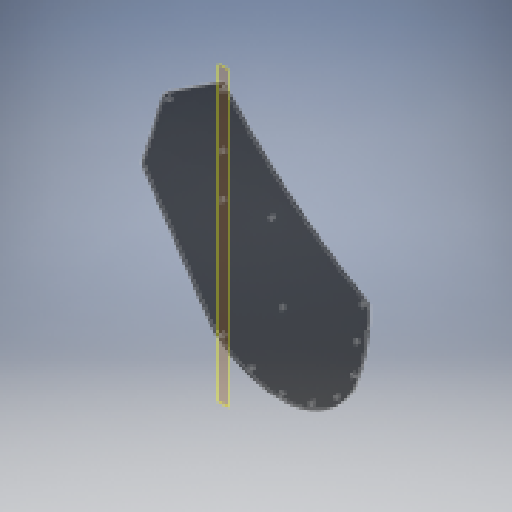
# Autodesk Inventor part: PolyIntakeSides
Saved by Autodesk Inventor 2026.1 (Build 301233000, 233)
## iProperties
Created: 2025-09-20
Part Number: PolyIntakeSides
Material: Polycarbonate, Smoke
Document SubType Name: Modeling
Designer: Teddy
Density: 1.2 g/cm^3
Appearance: Polycarbonate - Smoked
Author: Teddy
Autodesk Inventor part; units mm, degrees
ref_plane "YZ Plane" through (0, 0, 0) normal (1, 0, 0) x (0, 1, 0)
ref_plane "XZ Plane" through (0, 0, 0) normal (0, 1, 0) x (-1, 0, 0)
ref_plane "XY Plane" through (0, 0, 0) normal (0, 0, 1) x (1, 0, 0)
ref_plane "Work Plane1" through (0, 0, 0) normal (0, 0, 1) x (1, 0, 0)
sketch "Sketch1" plane through (0, 0, 0) normal (0, 0, 1) x (1, 0, 0)
  circle A0 centre (1.1684, 152.4) radius 2.0828 projected
  circle A1 centre (1.1684, 88.9) radius 2.1844 projected
  circle A2 centre (1.1684, 38.1) radius 2.1844 projected
  circle A3 centre (61.0614, 49.4192) radius 2.1844 projected
  circle A4 centre (1.1684, -101.6) radius 2.1844 projected
  circle A5 centre (169.7176, 13.9463) radius 2.1844 projected
  circle A6 centre (-62.568, 110.6374) radius 2.1844 projected
  arc A7 (-66.0482, 115.9488) -> (-68.6382, 112.5014) centre (-62.568, 110.6374) ccw
  arc A8 (5.9747, 156.5499) -> (-2.3118, 157.7114) centre (1.1684, 152.4) ccw
  arc A9 (171.6835, 7.9082) -> (176.0627, 14.1942) centre (169.7176, 13.9463) ccw construction
  circle A10 centre (61.0614, 49.4192) radius 6.35 construction
  circle A11 centre (1.1684, 88.9) radius 6.35 construction
  circle A12 centre (1.1684, 38.1) radius 6.35 construction
  arc A13 (-3.0452, -106.3506) -> (-2.7826, -106.5711) centre (1.1684, -101.6) ccw
  line L0 (-66.0482, 115.9488) -> (-2.3118, 157.7114)
  arc A14 (5.9747, 156.5499) -> (172.8551, 19.467) centre (486.6085, 571.5392) ccw
  circle A15 centre (72.9495, -37.5108) radius 2.286
  line L1 (-82.8745, 72.8532) -> (22.0714, -87.311) construction
  line L2 (-72.2491, -17.1807) -> (-105.9376, 34.2333) construction
  arc A16 (171.6835, 7.9082) -> (153.2328, 1.3335) centre (281.7757, -330.2205) ccw construction
  arc A17 (10.0948, -100.7846) -> (6.0913, -105.6109) centre (281.7757, -330.2205) ccw construction
  arc A18 (19.0893, -100.0694) -> (10.0948, -100.7846) centre (14.9463, -104.8817) ccw construction
  arc A19 (153.2328, 1.3335) -> (149.6297, -6.9388) centre (155.5282, -4.5871) ccw construction
  line L3 (12.9609, -192.1214) -> (40.8456, -173.8503) construction
  arc A20 (19.0893, -100.0694) -> (38.9783, -112.7468) centre (72.9495, -37.5108) ccw construction
  line L4 (281.7757, -330.2205) -> (72.9495, -37.5108) construction
  line L5 (40.8456, -173.8503) -> (129.0057, -116.0843) construction
  arc A21 (36.3651, -118.5342) -> (161.4679, -29.2829) centre (72.9495, -37.5108) ccw construction
  arc A22 (33.752, -124.3216) -> (75.4374, -132.7283) centre (72.9495, -37.5108) ccw construction
  arc A23 (39.5647, -113.0492) -> (33.752, -124.3216) centre (36.3651, -118.5342) ccw construction
  arc A24 (167.7906, -28.6951) -> (155.4015, -31.1592) centre (161.4679, -29.2829) ccw construction
  arc A25 (38.9783, -112.7468) -> (155.1451, -29.8706) centre (72.9495, -37.5108) ccw construction
  arc A26 (155.1451, -29.8706) -> (149.6297, -6.9388) centre (72.9495, -37.5108) ccw construction
  arc A27 (161.8616, -71.6749) -> (176.0627, 14.1942) centre (-39.6726, 5.7638) ccw
  arc A28 (161.8616, -71.6749) -> (167.7906, -28.6951) centre (72.9495, -37.5108) ccw construction
  arc A29 (176.0627, 14.1942) -> (172.8551, 19.467) centre (169.7176, 13.9463) ccw
  arc A30 (-2.7826, -106.5711) -> (75.4374, -132.7283) centre (72.286, -12.1194) ccw
  arc A31 (75.4374, -132.7283) -> (161.8616, -71.6749) centre (72.9495, -37.5108) ccw
  arc A32 (-2.7826, -106.5711) -> (6.0913, -105.6109) centre (1.1684, -101.6) ccw construction
  circle A33 centre (36.3651, -118.5342) radius 2.286
  circle A34 centre (72.4832, -126.4095) radius 2.286
  circle A35 centre (108.6819, -118.9135) radius 2.286
  circle A36 centre (138.7021, -97.3421) radius 2.286
  circle A37 centre (157.3531, -65.4254) radius 2.286
  circle A38 centre (161.41, -28.682) radius 2.286
  line L6 (-68.6382, 112.5014) -> (-92.7323, 34.0383)
  line L7 (-91.2146, 23.3498) -> (-16.2187, -91.1058)
  arc A39 (-16.2187, -91.1058) -> (-3.0452, -106.3506) centre (47.5176, -49.3432) ccw
  line L8 (-82.8745, 72.8532) -> (-83.8065, 69.8181) projected
  arc A40 (-92.7323, 34.0383) -> (-91.2146, 23.3498) centre (-80.5918, 30.3103) ccw
  point P0 (0, 0)
  point P1 (120.8923, -104.7118)
  point P2 (-94.4829, 28.3377)
  dimension "d0" = 12.7
  dimension "d3" = 635
  dimension "d6" = 4.572
  dimension "d10" = 355.6
  dimension "d11" = 355.6
  dimension "d12" = 6.35
  dimension "d13" = 69.85
  dimension "d14" = 165.1
  dimension "d15" = 13.97
  dimension "d17" = 6.35
  dimension "d18" = 25.4
  dimension "d19" = 25.4
  dimension "d21" = 215.9
  dimension "d22" = 120.65
  dimension "d23" = 4.572
  dimension "d26" = 120
  dimension "d28" = 6.35
  dimension "d29" = 76.2
  dimension "d30" = 12.7
  constraints: 54 point on circle, 34 centre point, 22 tangent, 12 end point, 10 coincident, 7 equal radius, 4 point on line, 3 parallel, 1 collinear, 12 other
  measures "d0" diameter of A7
  measures "d3" radius of A14
  measures "d6" diameter of A15
  measures "d10" radius of A16
  measures "d11" radius of A17
  measures "d12" radius of A18
  measures "d13" distance from line of L1 A15.centre
  measures "d14" diameter of A20
  measures "d15" distance of point (120.892, -104.712) L5.end
  measures "d17" radius of A23
  measures "d18" distance of A18.centre A21.start
  measures "d19" distance of A19.centre A21.end
  measures "d21" radius of A27
  measures "d22" radius of A30
  measures "d23" diameter of A33
  measures "d28" distance from line of L2 point (-94.483, 28.338)
  measures "d29" radius of A39
  measures "d30" radius of A40
extrude "Extrusion1" add sketch "Sketch1" along normal blind 3.175
body "Solid1"
